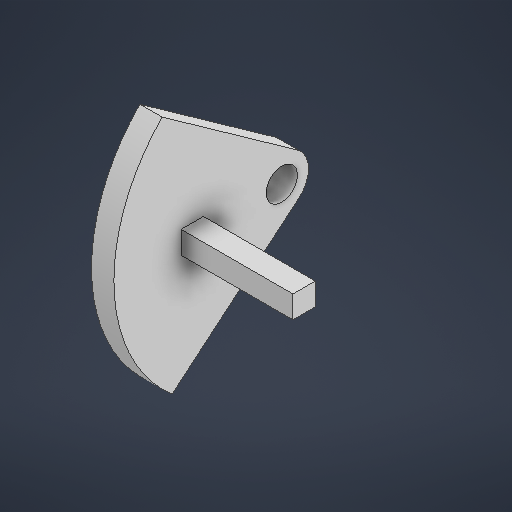
# Autodesk Inventor part: pitch gear v2
Saved by Autodesk Inventor 2026.2 (Build 302298000, 298)
## iProperties
Created: 2026-01-13
Part Number: pitch gear v2
Material: Generic
Document SubType Name: Modeling
Designer: User
Density: 1 g/cm^3
Appearance: Default
Author: User
Autodesk Inventor part; units mm, degrees
ref_plane "YZ Plane" through (0, 0, 0) normal (1, 0, 0) x (0, 1, 0)
ref_plane "XZ Plane" through (0, 0, 0) normal (0, 1, 0) x (-1, 0, 0)
ref_plane "XY Plane" through (0, 0, 0) normal (0, 0, 1) x (1, 0, 0)
sketch "Sketch1" plane through (0, 0, 0) normal (1, 0, 0) x (0, 1, 0)
  arc A0 (52.6508, 53.4125) -> (-56.7805, 48.9997) centre (0, 0) ccw
  circle A1 centre (0, 0) radius 7
  arc A2 (-9.1925, -7.7135) -> (9.1925, -7.7135) centre (0, 0) ccw
  line L0 (-9.1925, -7.7135) -> (-56.7805, 48.9997)
  line L1 (0, -37.4043) -> (0, 140.4256) projected
  line L2 (9.1925, -7.7135) -> (52.6508, 53.4125)
  point P0 (-112.1792, 115.0213)
  point P1 (112.1792, 115.0213)
  dimension "d0" = 150
  dimension "d1" = 14
  dimension "d2" = 5
  dimension "d3" = 40
  constraints: 4 end point, 4 point on circle, 3 centre point, 2 coincident, 2 symmetric about line, 1 tangent
  measures "d0" diameter of A0
  measures "d1" diameter of A1
  measures "d2" radial gap between concentric circles of A1 A2
  measures "d3" angle of L1 L0
extrude "Extrusion1" add sketch "Sketch1" along normal blind 10 contours L2 A2 L1 A1 A0 | L1 A1 A2 L0 A0
sketch "Sketch2" plane through (10, 0, 0) normal (1, 0, 0) x (0, 0, -1)
  line L0 (-35, -5.0063) -> (-45, -5.0063)
  line L1 (-45, -5.0063) -> (-45, 4.9937)
  line L2 (-45, 4.9937) -> (-35, 4.9937)
  line L3 (-35, 4.9937) -> (-35, -5.0063)
  point P0 (0, 0)
  dimension "d6" = 10
  dimension "d7" = 10
  dimension "d10" = 35
  constraints: 8 end point, 2 parallel, 1 horizontal, 1 perpendicular
  measures "d6" distance of L2.end L0.start
  measures "d7" distance of L1.end L2.end
  measures "d10" distance from line of L3 point (0, 0)
extrude "Extrusion2" add sketch "Sketch2" along normal blind 50
body "Solid1"
